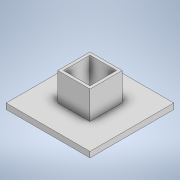
# Autodesk Inventor part: Motor_Key_Bearing_3_3
Saved by Autodesk Inventor 2022 (Build 260153000, 153)
## iProperties
Created: 2023-03-21
Part Number: Motor_Key_Bearing_3_3
Material: Generic
Document SubType Name: Modeling
Designer: zarek
Density: 1 g/cm^3
Appearance: Default
Author: zarek
Autodesk Inventor part; units mm, degrees
ref_plane "YZ Plane" through (0, 0, 0) normal (1, 0, 0) x (0, 1, 0)
ref_plane "XZ Plane" through (0, 0, 0) normal (0, 1, 0) x (-1, 0, 0)
ref_plane "XY Plane" through (0, 0, 0) normal (0, 0, 1) x (1, 0, 0)
sketch "Sketch1" plane through (0, 0, 0) normal (0, 1, 0) x (-1, 0, 0)
  line L0 (14.9, 14.9) -> (-14.9, 14.9)
  line L1 (-14.9, 14.9) -> (-14.9, -14.9)
  line L2 (-14.9, -14.9) -> (14.9, -14.9)
  line L3 (14.9, -14.9) -> (14.9, 14.9)
  point P0 (0, 0)
  dimension "d0" = 29.8
  dimension "d1" = 29.8
  dimension "d2" = 14.9
  dimension "d3" = 14.9
  constraints: 8 end point, 2 parallel, 1 horizontal, 1 perpendicular
  measures "d0" distance between parallel lines of L1 L3
  measures "d1" distance between parallel lines of L2 L0
  measures "d2" distance from line of L2 point (0, 0)
  measures "d3" distance from line of point (0, 0) L3
extrude "Extrusion1" add sketch "Sketch1" along normal blind 2
sketch "Sketch2" plane through (0, 2, 0) normal (0, 1, 0) x (1, 0, 0)
  line L0 (-5.715, -5.715) -> (5.715, -5.715)
  line L1 (5.715, -5.715) -> (5.715, 5.715)
  line L2 (5.715, 5.715) -> (-5.715, 5.715)
  line L3 (-5.715, 5.715) -> (-5.715, -5.715)
  line L4 (-4.715, -4.715) -> (4.715, -4.715)
  line L5 (4.715, -4.715) -> (4.715, 4.715)
  line L6 (4.715, 4.715) -> (-4.715, 4.715)
  line L7 (-4.715, 4.715) -> (-4.715, -4.715)
  line L8 (14.9, 14.9) -> (-14.9, 14.9) projected
  point P0 (0, 0)
  dimension "d6" = 11.43
  dimension "d7" = 11.43
  dimension "d8" = 5.715
  dimension "d9" = 5.715
  dimension "d10" = 1
  dimension "d11" = 1
  dimension "d12" = 1
  dimension "d13" = 1
  dimension "d18" = 9.185
  constraints: 16 end point, 4 parallel, 2 horizontal, 2 perpendicular
  measures "d6" distance between parallel lines of L2 L0
  measures "d7" distance between parallel lines of L1 L3
  measures "d8" distance from line of L3 point (0, 0)
  measures "d9" distance from line of L0 point (0, 0)
  measures "d10" distance between parallel lines of L2 L6
  measures "d11" distance between parallel lines of L3 L7
  measures "d12" distance between parallel lines of L0 L4
  measures "d13" distance between parallel lines of L1 L5
  measures "d18" distance between parallel lines of L2 L8
extrude "Extrusion2" add sketch "Sketch2" along normal blind 10
sketch "Sketch3" plane through (0, 2, 0) normal (0, 1, 0) x (1, 0, 0)
  line L0 (4.715, 4.715) -> (-4.715, 4.715) projected
  line L1 (4.715, -4.715) -> (4.715, 4.715) projected
  line L2 (-4.715, 4.715) -> (4.715, 4.715)
  line L3 (4.715, 4.715) -> (4.715, -4.715)
  line L4 (4.715, -4.715) -> (-4.715, -4.715)
  line L5 (-4.715, -4.715) -> (-4.715, 4.715)
  point P0 (0, 0)
  constraints: 8 end point, 2 parallel, 1 horizontal, 1 perpendicular
extrude "Extrusion3" cut sketch "Sketch3" against normal blind 10
equation "\"d1\" = d0"
equation "\"d2\" = 0.5 * d1"
equation "\"d3\" = 0.5 * d1"
equation "\"d7\" = d6"
equation "\"d8\" = 0.5 * d6"
equation "\"d9\" = 0.5 * d6"
body "Solid1"
